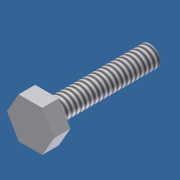
# Autodesk Inventor part: HW-00037
Saved by Autodesk Inventor 2012 (Build 160160000, 160)
## iProperties
Created: 2008-06-03
Part Number: HW-00037
Document SubType Name: Modeling
Designer: mcyr
Density: 1 g/cm^3
Description: Hex head bolt 5/16-18 x 1-1/4"
Mass: 0.962722 g
Surface Area: 6.85988 cm^2
Volume: 0.962722 cm^3
Material: Default
Title: HW-00012
Author: mcyr
Autodesk Inventor part; units mm, degrees
ref_plane "YZ Plane" through (0, 0, 0) normal (1, 0, 0) x (0, 1, 0)
ref_plane "XZ Plane" through (0, 0, 0) normal (0, 1, 0) x (-1, 0, 0)
ref_plane "XY Plane" through (0, 0, 0) normal (0, 0, 1) x (1, 0, 0)
sketch "Sketch1" plane through (0, 0, 0) normal (0, 0, 1) x (1, 0, 0)
  circle A0 centre (-0.6115, -1.5992) radius 3.175
  line L0 (-7.8705, -1.5992) -> (-4.241, 4.6873)
  line L1 (-4.241, 4.6873) -> (3.018, 4.6873)
  line L2 (3.018, 4.6873) -> (6.6475, -1.5992)
  line L3 (6.6475, -1.5992) -> (3.018, -7.8857)
  line L4 (3.018, -7.8857) -> (-4.241, -7.8857)
  line L5 (-4.241, -7.8857) -> (-7.8705, -1.5992)
  dimension "d10" = 12.573
  constraints: 12 end point, 1 centre point, 13 other
  measures "d10" distance between parallel lines of L4 L1
extrude "Extrusion1" add sketch "Sketch1" against normal blind 31.75 contours A0
extrude "Extrusion2" add sketch "Sketch1" along normal blind 5.08 contours A0 | L0 L1 L2 L3 L4 L5
thread "Thread1" size "5/16-18 UNC" class "2A" standard "ANSI Unified Screw Threads" full length
body "Solid1"
